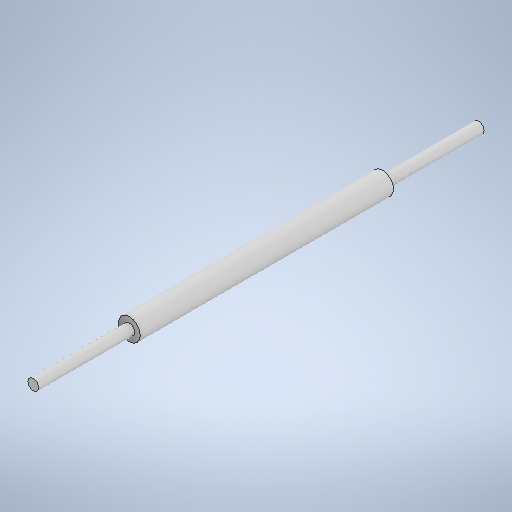
# Autodesk Inventor part: Main Shaft
Saved by Autodesk Inventor 2025.2 (Build 292293000, 293)
## iProperties
Created: 2025-02-15
Part Number: Main Shaft
Material: Generic
Document SubType Name: Modeling
Designer: shiva
Density: 1 g/cm^3
Appearance: Default
Author: shiva
Autodesk Inventor part; units mm, degrees
ref_plane "YZ Plane" through (0, 0, 0) normal (1, 0, 0) x (0, 1, 0)
ref_plane "XZ Plane" through (0, 0, 0) normal (0, 1, 0) x (-1, 0, 0)
ref_plane "XY Plane" through (0, 0, 0) normal (0, 0, 1) x (1, 0, 0)
sketch "Sketch1" plane through (0, 0, 0) normal (0, 0, 1) x (1, 0, 0)
  circle A0 centre (0, 0) radius 5
  circle A1 centre (0, 0) radius 2.5
  dimension "d0" = 10
  dimension "d1" = 5
  constraints: 2 centre point, 2 coincident
  measures "d0" diameter of A0
  measures "d1" diameter of A1
extrude "Extrusion1" add sketch "Sketch1" along normal blind 116 contours A0 | A1
extrude "Extrusion2" add sketch "Sketch1" along normal blind 44 from surface at 116 contours A1
extrude "Extrusion3" add sketch "Sketch1" against normal blind 44 contours A1
body "Solid1"
